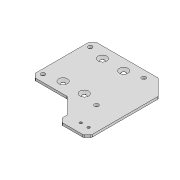
# Autodesk Inventor part: CCM_Mount_B
Saved by Autodesk Inventor 2020 (Build 240168000, 168)
## iProperties
Created: 2021-07-12
Part Number: CCM_Mount_B
Material: 一般
Document SubType Name: Modeling
Designer: magnarecta
Density: 1 g/cm^3
Appearance: 既定
Author: magnarecta
Autodesk Inventor part; units mm, degrees
ref_plane "YZ Plane" through (0, 0, 0) normal (1, 0, 0) x (0, 1, 0)
ref_plane "XZ Plane" through (0, 0, 0) normal (0, 1, 0) x (-1, 0, 0)
ref_plane "XY Plane" through (0, 0, 0) normal (0, 0, 1) x (1, 0, 0)
sketch "スケッチ1" plane through (0, 0, 0) normal (0, 1, 0) x (-1, 0, 0)
  line L0 (-40, -39) -> (40, -39)
  line L1 (40, -39) -> (40, 39)
  line L2 (40, 39) -> (-40, 39)
  line L3 (-40, 39) -> (-40, -39)
  line L4 (-40, -39) -> (40, 39) construction
  line L5 (40, -39) -> (-40, 39) construction
  point P0 (0, 0)
  dimension "d0" = 80
  dimension "d1" = 78
  constraints: 12 end point, 2 midpoint, 2 parallel, 1 horizontal, 1 perpendicular
  measures "d0" distance of L0.start L0.end
  measures "d1" distance of L0.end L1.end
extrude "押し出し1" add sketch "スケッチ1" along normal blind 3
sketch "スケッチ2" plane through (0, 3, 0) normal (0, 1, 0) x (1, 0, 0)
  line L0 (34, 30) -> (-34, 30)
  line L1 (-34, 30) -> (-34, -30)
  line L2 (-34, -30) -> (34, -30)
  line L3 (34, -30) -> (34, 30)
  line L4 (34, 30) -> (-34, -30) construction
  line L5 (-34, 30) -> (34, -30) construction
  point P0 (0, 0)
  dimension "d4" = 68
  dimension "d5" = 60
  constraints: 12 end point, 2 midpoint, 2 parallel, 1 horizontal, 1 perpendicular
  measures "d4" distance of L2.end L1.end
  measures "d5" distance of L1.end L0.end
hole "穴1" at (-34, 3, 30) at (34, 3, 30) at (34, 3, -30) at (-34, 3, -30) direction (0, -1, 0) diameter 5.2 depth 8 tip angle 118
sketch "スケッチ3" plane through (0, 3, 0) normal (0, 1, 0) x (1, 0, 0)
  line L0 (13.5, 25) -> (-13.5, 25)
  line L1 (-13.5, 25) -> (-13.5, -25)
  line L2 (-13.5, -25) -> (13.5, -25)
  line L3 (13.5, -25) -> (13.5, 25)
  line L4 (13.5, 25) -> (-13.5, -25) construction
  line L5 (-13.5, 25) -> (13.5, -25) construction
  point P0 (0, 0)
  dimension "d13" = 27
  dimension "d14" = 50
  constraints: 12 end point, 4 coincident, 2 midpoint, 2 parallel, 1 horizontal, 1 perpendicular
  measures "d13" distance of L0.start L0.end
  measures "d14" distance of L0.end L1.end
hole "穴2" at (-13.5, 3, 25) at (13.5, 3, 25) at (13.5, 3, -25) at (-13.5, 3, -25) direction (0, -1, 0) diameter 5.3 depth 8 tip angle 118 countersink diameter 11 countersink angle 90
sketch "スケッチ4" plane through (0, 0, 0) normal (0, -1, 0) x (1, 0, 0)
  line L0 (40, -39) -> (-40, -39) projected
  line L1 (26.3, -39) -> (63.5, -39)
  line L2 (63.5, -39) -> (63.5, 71)
  line L3 (63.5, 71) -> (26.3, 71)
  line L4 (26.3, 71) -> (26.3, -39)
  circle A0 centre (13.5, -25) radius 2.65 projected
  circle A1 centre (-13.5, 25) radius 2.65 projected
  circle A2 centre (13.5, 25) radius 2.65 projected
  circle A3 centre (-13.5, -25) radius 2.65 projected
  circle A4 centre (34, -30) radius 2.6 projected
  circle A5 centre (-34, 30) radius 2.6 projected
  circle A6 centre (34, 30) radius 2.6 projected
  circle A7 centre (-34, -30) radius 2.6 projected
  line L5 (-40, -39) -> (-40, 39) projected
  line L6 (40, -39) -> (-40, -39) projected
  line L7 (40, 39) -> (40, -39) projected
  line L8 (-40, 39) -> (40, 39) projected
  point P0 (0, 0)
  point P1 (26.3, 39)
  dimension "d23" = 110
  dimension "d24" = 50
  constraints: 8 end point, 2 parallel, 1 horizontal, 1 perpendicular, 1 point on line
  measures "d23" distance between parallel lines of L3 L0
  measures "d24" distance from line of L2 A0.centre
extrude "押し出し2" add sketch "スケッチ4" against normal up to surface (3 mm away) contours L7 L8 L4 L3 L2 L1
sketch "スケッチ5" plane through (0, 3, 0) normal (0, 1, 0) x (1, 0, 0)
  circle A0 centre (13.5, 25) radius 5.5 projected
  circle A1 centre (-13.5, -25) radius 5.5 projected
  circle A2 centre (13.5, -25) radius 5.5 projected
  circle A3 centre (-13.5, 25) radius 5.5 projected
  circle A4 centre (34, 30) radius 2.6 projected
  circle A5 centre (-34, -30) radius 2.6 projected
  circle A6 centre (34, -30) radius 2.6 projected
  circle A7 centre (-34, 30) radius 2.6 projected
  line L0 (63.5, 39) -> (63.5, -71) projected
  line L1 (-40, 39) -> (63.5, 39) projected
  line L2 (-40, 39) -> (-40, -39) projected
  line L3 (-40, -39) -> (26.3, -39) projected
  line L4 (26.3, -71) -> (26.3, -39) projected
  line L5 (63.5, -71) -> (26.3, -71) projected
  point P0 (0, 0)
  point P1 (53.5, -59.5)
  point P2 (43.5, -59.5)
  dimension "d28" = 10
  dimension "d29" = 11.5
  dimension "d30" = 10
  constraints: 1 horizontal alignment
  measures "d28" distance of point (43.5, -59.5) point (53.5, -59.5)
  measures "d29" distance from line of point (53.5, -59.5) L5
  measures "d30" distance from line of point (53.5, -59.5) L0
hole "穴3" at (53.5, 3, 59.5) at (43.5, 3, 59.5) direction (0, -1, 0) diameter 3.242 depth 11.8 tip angle 118 thread size "M4x0.7" class "6H" standard "ISO Metric profile"
chamfer "面取り1" distance 20 angle 45 2 edges at (63.5, 1.5, -39) (26.3, 1.5, 39)
chamfer "面取り2" distance 5 angle 45 4 edges at (63.5, 1.5, 71) (26.3, 1.5, 71) (-40, 1.5, 39) (-40, 1.5, -39)
fillet "フィレット3" radius 2 12 edges at (63.5, 1.5, 66) (58.5, 1.5, 71) (31.3, 1.5, 71) (26.3, 1.5, 66) (26.3, 1.5, 59) (6.3, 1.5, 39) (-35, 1.5, 39) (-40, 1.5, 34) (-40, 1.5, -34) (-35, 1.5, -39) (63.5, 1.5, -19) (43.5, 1.5, -39)
